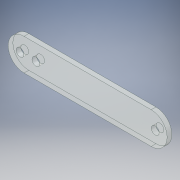
# Autodesk Inventor part: new acr connect
Saved by Autodesk Inventor 2019 (Build 230136000, 136)
## iProperties
Created: 2020-03-01
Part Number: new acr connect
Material: Glass
Document SubType Name: Modeling
Designer: KiranM
Density: 2.18 g/cm^3
Appearance: Clear
Author: KiranM
Autodesk Inventor part; units mm, degrees
ref_plane "YZ Plane" through (0, 0, 0) normal (1, 0, 0) x (0, 1, 0)
ref_plane "XZ Plane" through (0, 0, 0) normal (0, 1, 0) x (-1, 0, 0)
ref_plane "XY Plane" through (0, 0, 0) normal (0, 0, 1) x (1, 0, 0)
sketch "Sketch1" plane through (0, 0, 0) normal (0, 0, 1) x (1, 0, 0)
  line L0 (0, 0) -> (0, -20)
  line L1 (0, -20) -> (100, -20)
  line L2 (100, -20) -> (100, 0)
  line L3 (100, 0) -> (0, 0)
  line L4 (0, 0) -> (0, -10)
  line L5 (0, -10) -> (7.5, -10)
  circle A0 centre (7.5, -10) radius 2.5
  circle A1 centre (92.5, -10) radius 2.5
  dimension "d2" = 10
  dimension "d3" = 7.5
  dimension "d4" = 5
  dimension "d5" = 5
  dimension "d6" = 7.5
  constraints: 12 end point, 4 perpendicular, 2 centre point, 1 coincident, 1 midpoint, 1 vertical
  measures "d2" distance of L0.start L4.end
  measures "d3" distance of L4.end L5.end
  measures "d4" diameter of A0
  measures "d5" diameter of A1
  measures "d6" distance from line of A1.centre L2
extrude "Extrusion1" add sketch "Sketch1" along normal blind 3
fillet "Fillet1" radius 10 1 edges at (100, 0, 1.5)
fillet "Fillet2" radius 10 1 edges at (100, -20, 1.5)
fillet "Fillet3" radius 10 1 edges at (0, -20, 1.5)
fillet "Fillet4" radius 10 1 edges at (0, 0, 1.5)
sketch "Sketch2" plane through (0, 0, 0) normal (0, 0, -1) x (-1, 0, 0)
  circle A0 centre (-7.5, -10) radius 2.5 projected
  circle A1 centre (-17.5, -10) radius 2.5
  point P0 (0, 0)
  constraints: 1 centre point
extrude "Extrusion2" cut sketch "Sketch2" against normal through all contours A1
body "Solid1"
